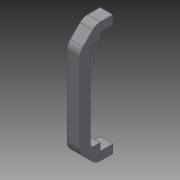
# Autodesk Inventor part: 27080914ServoMount
Saved by Autodesk Inventor 2016 (Build 200138000, 138)
## iProperties
Created: 2013-08-02
Part Number: 27080914ServoMount
Material: Generic
Document SubType Name: Modeling
Designer: Eric
Density: 1 g/cm^3
Appearance: Default
Author: Eric
Autodesk Inventor part; units mm, degrees
ref_plane "YZ Plane" through (0, 0, 0) normal (1, 0, 0) x (0, 1, 0)
ref_plane "XZ Plane" through (0, 0, 0) normal (0, 1, 0) x (-1, 0, 0)
ref_plane "XY Plane" through (0, 0, 0) normal (0, 0, 1) x (1, 0, 0)
sketch "Sketch1" plane through (0, 0, 0) normal (1, 0, 0) x (0, 1, 0)
  line L0 (48.5, 0) -> (52.5, 0)
  line L1 (52.5, 0) -> (52.5, 8)
  line L2 (-4, 8) -> (-4, 0)
  line L3 (-4, 0) -> (0, 0)
  line L4 (0, 0) -> (0, 6)
  line L5 (4.5, 10.5) -> (44, 10.5)
  line L6 (48.5, 6) -> (48.5, 0)
  line L7 (3.5, 15.5) -> (45, 15.5)
  line L8 (45, 15.5) -> (52.5, 8)
  line L9 (-4, 8) -> (3.5, 15.5)
  line L10 (48.5, 6) -> (45, 6)
  line L11 (45, 6) -> (45, 9.5)
  line L12 (0, 6) -> (3.5, 6)
  line L13 (3.5, 6) -> (3.5, 9.5)
  arc A0 (45, 9.5) -> (44, 10.5) centre (44, 9.5) ccw
  arc A1 (4.5, 10.5) -> (3.5, 9.5) centre (4.5, 9.5) ccw
  point P0 (0, 0)
  point P1 (24.25, 15.5)
  point P2 (24.25, 10.5)
  dimension "d4" = 48.5
  dimension "d31" = 5
  dimension "d37" = 4
  dimension "d46" = 3.5
  dimension "d48" = 1
  dimension "d50" = 8
  dimension "d51" = 4.5
  dimension "d52" = 6
  constraints: 28 end point, 5 equal length, 4 perpendicular, 4 point on circle, 4 tangent, 3 horizontal, 3 vertical, 2 centre point, 2 coincident, 2 midpoint, 2 vertical alignment, 1 equal radius, 1 horizontal alignment, 1 parallel
  measures "d4" distance between parallel lines of L6 L4
  measures "d31" distance between parallel lines of L5 L7
  measures "d37" distance of L0.start L0.end
  measures "d46" distance of L6.start L10.end
  measures "d48" radius of A0
  measures "d50" distance of L0.end L1.end
  measures "d51" distance between parallel lines of L5 L12
  measures "d52" distance of L3.end L4.end
extrude "Extrusion1" add sketch "Sketch1" along normal blind 6
fillet "Fillet1" radius 5 4 edges at (3, 3.5, 15.5) (3, 45, 15.5) (3, 52.5, 8) (3, -4, 8)
equation "\"d4\" = ServoMount"
equation "\"ServoMountLength\" = 48.5"
equation "\"ServoMount\" = 48.5"
body "Solid1"
